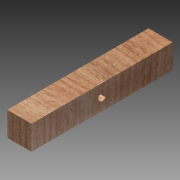
# Autodesk Inventor part: CNC-1.1v-X-7-( axis mover nut inside)
Saved by Autodesk Inventor 2015 (Build 190159000, 159)
## iProperties
Created: 2015-07-14
Part Number: CNC-1.1v-X-7-( axis mover nut inside)
Material: Generic
Document SubType Name: Modeling
Designer: Bangladesh
Density: 1 g/cm^3
Appearance: Default
Author: Bangladesh
Autodesk Inventor part; units mm, degrees
ref_plane "YZ Plane" through (0, 0, 0) normal (1, 0, 0) x (0, 1, 0)
ref_plane "XZ Plane" through (0, 0, 0) normal (0, 1, 0) x (-1, 0, 0)
ref_plane "XY Plane" through (0, 0, 0) normal (0, 0, 1) x (1, 0, 0)
sketch "Sketch1" plane through (0, 0, 0) normal (0, 1, 0) x (-1, 0, 0)
  line L0 (19.05, 111.1) -> (-19.05, 111.1)
  line L1 (-19.05, 111.1) -> (-19.05, -111.1)
  line L2 (-19.05, -111.1) -> (19.05, -111.1)
  line L3 (19.05, -111.1) -> (19.05, 111.1)
  line L4 (19.05, 111.1) -> (-19.05, -111.1) construction
  line L5 (-19.05, 111.1) -> (19.05, -111.1) construction
  point P0 (0, 0)
  dimension "d0" = 222.2
  dimension "d1" = 38.1
  constraints: 12 end point, 2 midpoint, 2 parallel, 1 horizontal, 1 perpendicular
  measures "d0" distance of L2.end L0.start
  measures "d1" distance of L1.end L2.end
extrude "Extrusion1" add sketch "Sketch1" along normal mid plane 38.1
sketch "Sketch2" plane through (19.05, -19.05, -111.1) normal (1, 0, 0) x (0, 0, -1)
  circle A0 centre (-111.1, 19.05) radius 6.619
  line L0 (-111.1, 12.431) -> (-116.8323, 15.7405)
  line L1 (-116.8323, 15.7405) -> (-116.8323, 22.3595)
  line L2 (-116.8323, 22.3595) -> (-111.1, 25.669)
  line L3 (-111.1, 25.669) -> (-105.3677, 22.3595)
  line L4 (-105.3677, 22.3595) -> (-105.3677, 15.7405)
  line L5 (-105.3677, 15.7405) -> (-111.1, 12.431)
  dimension "d4" = 13.2381
  constraints: 12 end point, 2 coincident, 1 vertical alignment, 15 other
extrude "Extrusion2" cut sketch "Sketch2" against normal through all contours L4 L5 L0 L1 L2 L3
body "Solid1"
